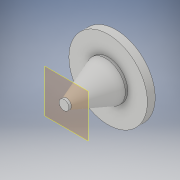
# Autodesk Inventor part: Aerospike base
Saved by Autodesk Inventor 2017 (Build 210142000, 142)
## iProperties
Created: 2016-10-16
Part Number: Aerospike base
Material: Generic
Document SubType Name: Modeling
Designer: Will
Density: 1 g/cm^3
Appearance: Default
Author: Will
Autodesk Inventor part; units mm, degrees
ref_plane "YZ Plane" through (0, 0, 0) normal (1, 0, 0) x (0, 1, 0)
ref_plane "XZ Plane" through (0, 0, 0) normal (0, 1, 0) x (-1, 0, 0)
ref_plane "XY Plane" through (0, 0, 0) normal (0, 0, 1) x (1, 0, 0)
sketch "Sketch1" plane through (0, 0, 0) normal (0, 0, 1) x (1, 0, 0)
  circle A0 centre (0, 0) radius 12.7
  dimension "d0" = 25.4
  constraints: 1 centre point, 1 coincident
  measures "d0" diameter of A0
extrude "Extrusion1" add sketch "Sketch1" along normal blind 1.5875
ref_plane "Work Plane1" through (0, 0, 26.9875) normal (0, 0, 1) x (1, 0, 0)
sketch "Sketch2" plane through (0, 0, 26.9875) normal (0, 0, 1) x (1, 0, 0)
  circle A0 centre (0, 0) radius 3.175
  dimension "d4" = 6.35
  constraints: 1 centre point, 1 coincident
  measures "d4" diameter of A0
extrude "Extrusion2" add sketch "Sketch2" along normal blind 1.5875
loft "Loft1" add section 1 edges at (-12.7, 0, 1.5875) section 2 edges at (-3.175, 0, 26.9875)
sketch "Sketch3" plane through (0, 0, 0) normal (0, 0, -1) x (-1, 0, 0)
  circle A0 centre (0, 0) radius 25.4
  dimension "d11" = 50.8
  constraints: 1 centre point, 1 coincident
  measures "d11" diameter of A0
extrude "Extrusion3" add sketch "Sketch3" along normal blind 5.08
sketch "Sketch5" plane through (0, 0, -5.08) normal (0, 0, -1) x (-1, 0, 0)
  point P0 (0, 0)
body "Solid1"
